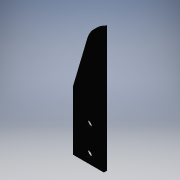
# Autodesk Inventor part: 16in coil holder plate
Saved by Autodesk Inventor 2016 (Build 200138000, 138)
## iProperties
Created: 2016-02-02
Part Number: 16in coil holder plate
Material: UHMW, Black
Document SubType Name: Modeling
Designer: Scott
Density: 0.94 g/cm^3
Appearance: Smooth - Black
Author: Scott
Autodesk Inventor part; units mm, degrees
ref_plane "YZ Plane" through (0, 0, 0) normal (1, 0, 0) x (0, 1, 0)
ref_plane "XZ Plane" through (0, 0, 0) normal (0, 1, 0) x (-1, 0, 0)
ref_plane "XY Plane" through (0, 0, 0) normal (0, 0, 1) x (1, 0, 0)
sketch "Sketch1" plane through (0, 0, 0) normal (0, 0, 1) x (1, 0, 0)
  line L0 (-114.3, 77.8543) -> (-127, 77.8543) projected
  line L1 (-127, 77.8543) -> (-163.2323, 36.0005) projected
  arc A0 (-163.2323, 36.0005) -> (-215.9, -105.3078) centre (0, -105.3078) ccw projected
  line L2 (-152.4, -105.3078) -> (-215.9, -105.3078) projected
  arc A1 (152.4, -105.3078) -> (-152.4, -105.3078) centre (0, -105.3078) ccw projected
  line L3 (215.9, -105.3078) -> (152.4, -105.3078) projected
  arc A2 (215.9, -105.3078) -> (163.2323, 36.0005) centre (0, -105.3078) ccw projected
  line L4 (163.2323, 36.0005) -> (127, 77.8543) projected
  line L5 (127, 77.8543) -> (114.3, 77.8543) projected
  line L6 (114.3, 77.8543) -> (114.3, 90.5543) projected
  line L7 (114.3, 90.5543) -> (46.5518, 105.5138) projected
  arc A3 (46.5518, 105.5138) -> (-46.5518, 105.5138) centre (0, -105.3078) ccw projected
  line L8 (-46.5518, 105.5138) -> (-114.3, 90.5543) projected
  line L9 (-114.3, 90.5543) -> (-114.3, 77.8543) projected
  circle A4 centre (-174.6359, -42.9949) radius 3.302 projected
  circle A5 centre (-181.5133, -67.4461) radius 3.302 projected
  circle A6 centre (-184.9846, -92.6078) radius 3.302 projected
  circle A7 centre (-12.7, 63.1241) radius 3.302 projected
  circle A8 centre (-37.8617, 76.2055) radius 3.302 projected
  circle A9 centre (-62.0706, 51.784) radius 3.302 projected
  circle A10 centre (12.7, 63.1241) radius 3.302 projected
  circle A11 centre (62.0706, 51.784) radius 3.302 projected
  circle A12 centre (62.3129, 69.3281) radius 3.302 projected
  circle A13 centre (174.6359, -42.9949) radius 3.302 projected
  circle A14 centre (164.6231, -67.4949) radius 3.302 projected
  circle A15 centre (181.5133, -67.4461) radius 3.302 projected
  circle A16 centre (184.9846, -92.6078) radius 3.302 projected
  circle A17 centre (168.4319, -92.6078) radius 3.302 projected
  circle A18 centre (157.0918, -43.2372) radius 3.302 projected
  circle A19 centre (37.8617, 76.2055) radius 3.302 projected
  circle A20 centre (37.8128, 59.3154) radius 3.302 projected
  circle A21 centre (12.7, 79.6768) radius 3.302 projected
  circle A22 centre (-62.3129, 69.3281) radius 3.302 projected
  circle A23 centre (-37.8128, 59.3154) radius 3.302 projected
  circle A24 centre (-12.7, 79.6768) radius 3.302 projected
  circle A25 centre (-168.4319, -92.6078) radius 3.302 projected
  circle A26 centre (-164.6231, -67.4949) radius 3.302 projected
  circle A27 centre (-157.0918, -43.2372) radius 3.302 projected
  line L10 (-127, 143.7166) -> (-127, -105.3078) projected
  line L11 (-127, -21.0655) -> (-127, 108.4537)
  line L12 (-142.24, -21.0655) -> (-142.24, 38.6612) construction
  circle A28 centre (-142.24, -7.2274) radius 3.302
  circle A29 centre (-142.24, 18.1726) radius 3.302
  line L13 (-157.48, -21.0655) -> (-157.48, 42.6453)
  line L14 (-127, -21.0655) -> (-157.48, -21.0655)
  line L15 (-127, 108.4537) -> (-131.3752, 105.9825)
  line L16 (-143.2518, 91.0321) -> (-157.48, 42.6453)
  arc A30 (-131.3752, 105.9825) -> (-143.2518, 91.0321) centre (-118.8834, 83.8665) ccw
  circle A31 centre (142.24, 14.8706) radius 3.302 projected
  circle A32 centre (-142.24, 14.8706) radius 3.302 projected
  circle A33 centre (-142.24, -10.5294) radius 3.302 projected
  circle A34 centre (142.24, -10.5294) radius 3.302 projected
  point P0 (0, 0)
  dimension "d1" = 6.604
  dimension "d2" = 6.604
  dimension "d3" = 25.4
  dimension "d6" = 15.24
  dimension "d7" = 15.24
  dimension "d8" = 25.4
  constraints: 13 end point, 5 point on line, 3 centre point, 3 point on circle, 2 tangent, 2 vertical, 1 perpendicular, 1 vertical alignment, 1 other
  measures "d1" diameter of A28
  measures "d2" diameter of A29
  measures "d3" distance of A29.centre A28.centre
  measures "d6" distance between parallel lines of L12 L13
  measures "d7" distance between parallel lines of L11 L12
  measures "d8" radius of A30
extrude "Extrusion1" add sketch "Sketch1" along normal blind 3.175 contours L10 L14 L13 L1 | L1 L16 A30 L15 L10 | A28 A33 | A29 A32 picked at (-142.4059, -12.7065) picked at (-142.4059, 12.6935)
sketch "Sketch2" plane through (0, 0, 0) normal (0, 0, -1) x (-1, 0, 0)
  line L0 (127, -21.0655) -> (127, 108.4537) projected
  line L1 (157.48, 42.6453) -> (157.48, -21.0655) projected
  line L2 (127, -21.0655) -> (157.48, -21.0655)
  line L3 (157.48, -21.0655) -> (157.48, -15.2234)
  line L4 (157.48, -15.2234) -> (127, -15.2234)
  line L5 (127, -15.2234) -> (127, -21.0655)
  point P0 (0, 0)
  constraints: 8 end point, 2 parallel, 1 horizontal, 1 perpendicular, 1 point on line
extrude "Extrusion2" cut sketch "Sketch2" against normal blind 25.4
body "Solid1"
